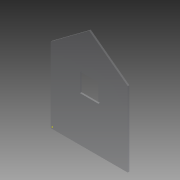
# Autodesk Inventor part: fundo
Saved by Autodesk Inventor 2015 (Build 190159000, 159)
## iProperties
Created: 2016-08-07
Part Number: fundo
Material: Polycarbonate, Clear
Document SubType Name: Modeling
Designer: Gabriel
Density: 1.2 g/cm^3
Appearance: Polycarbonate - Clear
Author: Gabriel
Autodesk Inventor part; units mm, degrees
ref_plane "YZ Plane" through (0, 0, 0) normal (1, 0, 0) x (0, 1, 0)
ref_plane "XZ Plane" through (0, 0, 0) normal (0, 1, 0) x (-1, 0, 0)
ref_plane "XY Plane" through (0, 0, 0) normal (0, 0, 1) x (1, 0, 0)
sketch "Sketch1" plane through (0, 0, 0) normal (0, 0, 1) x (1, 0, 0)
  point P0 (0, 0)
sketch "Sketch2" plane through (0, 0, 0) normal (0, 0, 1) x (1, 0, 0)
  line L0 (0, 0) -> (335, 0)
  line L1 (335, 0) -> (335, 450)
  line L2 (335, 450) -> (0, 450)
  line L3 (0, 450) -> (0, 0)
  line L4 (0, 0) -> (167.5, 0)
  dimension "d0" = 335
  dimension "d1" = 450
  dimension "d2" = 167.5
  constraints: 10 end point, 2 parallel, 1 horizontal, 1 midpoint, 1 perpendicular
  measures "d0" distance of L2.end L1.end
  measures "d1" distance of L1.end L0.end
  measures "d2" distance of L0.start L4.end
extrude "Extrusion1" add sketch "Sketch2" along normal blind 7
sketch "Sketch3" plane through (0, 0, 7) normal (0, 0, 1) x (1, 0, 0)
  line L0 (0, 0) -> (167.5, 0)
  line L1 (0, 0) -> (335, 0) projected
  line L2 (167.5, 0) -> (167.5, 450)
  line L3 (335, 450) -> (0, 450) projected
  line L4 (0, 0) -> (0, 325)
  line L5 (0, 450) -> (0, 0) projected
  line L6 (0, 325) -> (335, 325)
  line L7 (335, 0) -> (335, 450) projected
  line L8 (335, 325) -> (167.5, 450)
  line L9 (167.5, 450) -> (0, 325)
  dimension "d5" = 167.5
  dimension "d6" = 325
  constraints: 12 end point, 2 midpoint, 2 point on line, 1 perpendicular
  measures "d5" distance of L0.start L0.end
  measures "d6" distance of L0.start L4.end
extrude "Extrusion2" cut sketch "Sketch3" against normal blind 166.0375 contours L5 L3 L9
sketch "Sketch5" plane through (0, 0, 7) normal (0, 0, 1) x (1, 0, 0)
  line L0 (167.5, 450) -> (335, 450)
  line L1 (335, 450) -> (167.5, 450) projected
  line L2 (335, 450) -> (335, 0)
  line L3 (335, 0) -> (335, 450) projected
  line L4 (335, 0) -> (335, 325)
  line L5 (167.5, 450) -> (335, 325)
  line L6 (335, 450) -> (167.5, 450)
  line L7 (335, 325) -> (335, 450)
  point P0 (0, 0)
  dimension "d10" = 325
  constraints: 12 end point, 4 collinear, 1 point on line
  measures "d10" distance of L2.end L4.end
extrude "Extrusion3" cut sketch "Sketch5" against normal blind 305.45
sketch "Sketch9" plane through (0, 0, 7) normal (0, 0, 1) x (1, 0, 0)
  line L0 (0, 325) -> (335, 325)
  line L1 (335, 325) -> (167.5, 325)
  line L2 (167.5, 325) -> (167.5, 275)
  line L3 (167.5, 275) -> (207.5, 275)
  line L4 (207.5, 275) -> (127.5, 275)
  line L5 (127.5, 275) -> (127.5, 195)
  line L6 (127.5, 195) -> (207.5, 195)
  line L7 (207.5, 195) -> (207.5, 275)
  point P0 (0, 0)
  dimension "d20" = 50
  dimension "d21" = 40
  dimension "d22" = 80
  dimension "d23" = 80
  dimension "d24" = 80
  constraints: 16 end point, 4 perpendicular, 1 horizontal, 1 midpoint, 1 point on line
  measures "d20" distance of L1.end L2.end
  measures "d21" distance of L2.end L3.end
  measures "d22" distance of L3.end L4.end
  measures "d23" distance of L4.end L5.end
  measures "d24" distance of L5.end L6.end
extrude "Extrusion5" cut sketch "Sketch9" against normal blind 10
body "Solid1"
